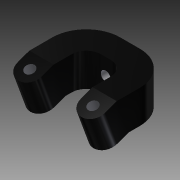
# Autodesk Inventor part: MountC
Saved by Autodesk Inventor 2015 (Build 190159000, 159)
## iProperties
Created: 2017-01-08
Part Number: MountC
Material: Generic
Document SubType Name: Modeling
Designer: Ernest
Density: 1 g/cm^3
Appearance: Default
Mass: 135.561 g
Surface Area: 237.117 cm^2
Volume: 135.561 cm^3
Author: Ernest
Autodesk Inventor part; units mm, degrees
ref_plane "YZ Plane" through (0, 0, 0) normal (1, 0, 0) x (0, 1, 0)
ref_plane "XZ Plane" through (0, 0, 0) normal (0, 1, 0) x (-1, 0, 0)
sketch "Sketch1" plane through (0, 0, 0) normal (0, 0, 1) x (1, 0, 0)
  circle A0 centre (0, 0) radius 5
  circle A1 centre (65, 0) radius 5
  circle A2 centre (0, 0) radius 12.5
  circle A3 centre (65, 0) radius 12.5
  line L0 (22.5, 9.5) -> (42.5, 9.5)
  line L1 (42.5, 9.5) -> (42.5, -10.5)
  line L2 (42.5, -10.5) -> (22.5, -10.5)
  line L3 (22.5, -10.5) -> (22.5, 9.5)
  line L4 (0, 0) -> (65, 0) construction
  line L5 (32.5, 0) -> (32.5, 40) construction
  line L6 (27.5, 40) -> (37.5, 40)
  line L7 (12.5, 0) -> (12.5, 25)
  line L8 (52.5, 0) -> (52.5, 25)
  arc A4 (27.5, 40) -> (12.5, 25) centre (27.5, 25) ccw
  arc A5 (52.5, 25) -> (37.5, 40) centre (37.5, 25) ccw
  line L9 (-12.5, 0) -> (-12.5, 30)
  line L10 (77.5, 0) -> (77.5, 30)
  line L11 (22.5, 65) -> (42.5, 65)
  arc A6 (22.5, 65) -> (-12.5, 30) centre (22.5, 30) ccw
  arc A7 (77.5, 30) -> (42.5, 65) centre (42.5, 30) ccw
  point P0 (22.5, 40)
  point P1 (42.5, 40)
  dimension "d0" = 10
  dimension "d1" = 10
  dimension "d2" = 65
  dimension "d3" = 25
  dimension "d4" = 25
  dimension "d5" = 22.5
  dimension "d6" = 22.5
  dimension "d7" = 9.5
  dimension "d8" = 10.5
  dimension "d11" = 20
  dimension "d12" = 10
  dimension "d13" = 40
  dimension "d14" = 15
  dimension "d15" = 65
  dimension "d16" = 35
  constraints: 24 end point, 12 point on circle, 12 tangent, 8 centre point, 4 horizontal, 4 point on line, 3 coincident, 3 perpendicular, 3 vertical, 2 equal radius, 2 midpoint, 2 parallel
  measures "d0" diameter of A0
  measures "d1" diameter of A1
  measures "d2" distance of A1.centre point (0, 0)
  measures "d3" diameter of A2
  measures "d4" diameter of A3
  measures "d5" distance from line of L3 point (0, 0)
  measures "d6" distance from line of L1 A1.centre
  measures "d7" distance from line of L0 point (0, 0)
  measures "d8" distance from line of point (0, 0) L2
  measures "d11" distance of point (22.5, 40) point (42.5, 40)
  measures "d12" distance of L5.end point (22.5, 40)
  measures "d13" distance of L5.start L5.end
  measures "d14" radius of A4
  measures "d15" distance from line of L11 L5.start
  measures "d16" radius of A6
extrude "Extrusion1" add sketch "Sketch1" along normal blind 34 contours A0 | A1 | A2 | A2 L9 A6 L11 A7 L10 A3 L8 A5 L6 A4 L7 | A3
ref_plane "Work Plane4" through (42.5, 65, 0) normal (0, 0.342, -0.9397) x (-1, 0, 0)
sketch "Sketch17" plane through (42.5, 65, 0) normal (0, 0.342, -0.9397) x (-1, 0, 0)
  ellipse E0 centre (42.5, -49.4513) end of major axis (30, -49.4513) minor radius 11.7462 (30, -49.4513) -> (55, -49.4513) ccw projected
  line L0 (30, -49.4513) -> (30, -25.959) projected
  ellipse E1 centre (15, -25.959) end of major axis (30, -25.959) minor radius 14.0954 (30, -25.959) -> (15, -11.8636) ccw projected
  line L1 (15, -11.8636) -> (5, -11.8636) projected
  ellipse E2 centre (5, -25.959) end of major axis (20, -25.959) minor radius 14.0954 (5, -11.8636) -> (-10, -25.959) ccw projected
  line L2 (-10, -25.959) -> (-10, -49.4513) projected
  ellipse E3 centre (-22.5, -49.4513) end of major axis (-35, -49.4513) minor radius 11.7462 (-35, -49.4513) -> (-10, -49.4513) ccw projected
  line L3 (-35, -49.4513) -> (-35, -21.2606) projected
  ellipse E4 centre (0, -21.2606) end of major axis (-35, -21.2606) minor radius 32.8892 (0, 11.6287) -> (-35, -21.2606) ccw projected
  line L4 (0, 11.6287) -> (20, 11.6287) projected
  ellipse E5 centre (20, -21.2606) end of major axis (55, -21.2606) minor radius 32.8892 (55, -21.2606) -> (20, 11.6287) ccw projected
  line L5 (55, -21.2606) -> (55, -49.4513) projected
  circle A0 centre (-22.5, -56.1975) radius 5
  circle A1 centre (42.5, -56.1975) radius 5
  circle A2 centre (-22.5, -56.1975) radius 12.5
  circle A3 centre (42.5, -56.1975) radius 12.5
  point P0 (42.5, -61.08)
  dimension "d83" = 10
  dimension "d84" = 10
  dimension "d85" = 25
  dimension "d86" = 25
  constraints: 4 centre point, 2 coincident, 8 other
  measures "d83" diameter of A0
  measures "d84" diameter of A1
  measures "d85" diameter of A2
  measures "d86" diameter of A3
extrude "Extrusion21" cut sketch "Sketch17" against normal blind 75.25 contours A1 | A0
extrude "Extrusion22" add sketch "Sketch17" against normal blind 58 contours A3 E0 | E0 A3 | A2 E3 | E3 A2
extrude "Extrusion23" cut sketch "Sketch17" against normal blind 15.9044 contours A3 E0 | E0 A3 | A2 E3 | E3 A2
sketch "Sketch19" plane through (65, 6.752, -4.2754) normal (0, 0.342, -0.9397) x (-1, 0, 0)
  circle A0 centre (0, 0) radius 5 projected
  circle A1 centre (0, 0) radius 12.5 projected
  circle A2 centre (65, 0) radius 5 projected
  circle A3 centre (65, 0) radius 12.5 projected
  line L0 (-12.5, 0) -> (-17.2667, 0)
  line L1 (-17.2667, 0) -> (-17.2667, -28.7026)
  line L2 (-17.2667, -28.7026) -> (21.0012, -28.7026)
  line L3 (21.0012, -28.7026) -> (21.0012, 0)
  line L4 (21.0012, 0) -> (12.5, 0)
  line L5 (52.5, 0) -> (49.0235, 0)
  line L6 (49.0235, 0) -> (49.0235, -27.0388)
  line L7 (49.0235, -27.0388) -> (85.6276, -27.0388)
  line L8 (85.6276, -27.0388) -> (85.6276, 0)
  line L9 (85.6276, 0) -> (77.5, 0)
  circle A4 centre (0, 0) radius 12.5
  circle A5 centre (65, 0) radius 12.5
  line L10 (-12.5, 0) -> (-12.5, 6.7462) projected
  line L11 (-12.5, -4.8825) -> (-12.5, 0) projected
  line L12 (-12.5, -4.8825) -> (-12.5, 0) projected
  line L13 (-12.5, 0) -> (-12.5, 23.3083) projected
  line L14 (-12.5, 23.3083) -> (-12.5, 34.9369) projected
  line L15 (-12.5, 6.7462) -> (-12.5, 34.9369) projected
  line L16 (77.5, 34.9369) -> (77.5, 6.7462) projected
  line L17 (77.5, 23.3083) -> (77.5, 34.9369) projected
  line L18 (77.5, 23.3083) -> (77.5, 0) projected
  line L19 (77.5, 0) -> (77.5, -4.8825) projected
  line L20 (77.5, -4.8825) -> (77.5, 0) projected
  line L21 (77.5, 0) -> (77.5, 6.7462) projected
  circle A6 centre (0, 0) radius 5 projected
  line L22 (12.5, 30.2385) -> (12.5, 6.7462) projected
  line L23 (12.5, 18.6098) -> (12.5, 30.2385) projected
  line L24 (12.5, 18.6098) -> (12.5, 0) projected
  line L25 (12.5, 0) -> (12.5, -4.8825) projected
  line L26 (12.5, -4.8825) -> (12.5, 0) projected
  line L27 (12.5, 0) -> (12.5, 6.7462) projected
  line L28 (52.5, 0) -> (52.5, 6.7462) projected
  line L29 (52.5, -4.8825) -> (52.5, 0) projected
  line L30 (52.5, -4.8825) -> (52.5, 0) projected
  line L31 (52.5, 0) -> (52.5, 18.6098) projected
  line L32 (52.5, 18.6098) -> (52.5, 30.2385) projected
  line L33 (52.5, 6.7462) -> (52.5, 30.2385) projected
  line L34 (-12.5, 0) -> (-12.5, 23.3083) projected
  line L35 (-12.5, 15.1562) -> (-12.5, -17.0681)
  line L36 (-12.5, -17.0681) -> (12.5, -17.0681)
  line L37 (12.5, -17.0681) -> (12.5, 15.1562)
  line L38 (12.5, 18.6098) -> (12.5, 0) projected
  line L39 (12.5, 15.1562) -> (-12.5, 15.1562)
  line L40 (52.5, 0) -> (52.5, 18.6098) projected
  line L41 (52.5, 15.1562) -> (52.5, -18.9753)
  line L42 (52.5, -18.9753) -> (77.5, -18.9753)
  line L43 (77.5, -18.9753) -> (77.5, 15.1562)
  line L44 (77.5, 23.3083) -> (77.5, 0) projected
  line L45 (77.5, 15.1562) -> (52.5, 15.1562)
  point P0 (65, -4.8825)
  point P1 (-12.5, 12.5)
  point P2 (-12.5, 5.9839)
  point P3 (77.5, 5.9839)
  point P4 (77.5, 12.5)
  point P5 (12.5, 5.9839)
  point P6 (12.5, 12.5)
  point P7 (52.5, 12.5)
  point P8 (52.5, 5.9839)
  constraints: 36 end point, 13 point on line, 10 perpendicular, 2 centre point, 2 coincident, 2 point on circle, 1 concentric, 1 horizontal
extrude "Extrusion29" add sketch "Sketch19" against normal blind 36.087 contours L25 L37 L36 L35 L11 A1 | A1 L10 L13 L39 L22 L24 | L19 L43 L42 L41 L29 A3 | A3 L28 L31 L45 L16 L18
extrude "Extrusion25" cut sketch "Sketch19" against normal blind 107.25 contours L25 L37 L36 L35 L11 A1 | L4 L3 L2 L1 L0 L11 L35 L36 L37 L25 | L19 L43 L42 L41 L29 A3 | L9 L8 L7 L6 L5 L29 L41 L42 L43 L19
sketch "Sketch20" plane through (22.5, 65, 0) normal (0, 1, 0) x (1, 0, 0)
  line L0 (20, 0) -> (0, 0) projected
  line L1 (0, 0) -> (0, -34) projected
  line L2 (20, -34) -> (0, -34) projected
  line L3 (20, 0) -> (20, -34) projected
  circle A0 centre (10, -17) radius 5
  point P0 (-22.5, 0)
  dimension "d97" = 10
  dimension "d98" = 20
  dimension "d99" = 34
  dimension "d100" = 17
  dimension "d101" = 10
  constraints: 1 centre point
  measures "d97" diameter of A0
  measures "d98" distance of L0.start L0.end
  measures "d99" distance of L0.end L1.end
  measures "d100" distance from line of L0 A0.centre
  measures "d101" distance from line of L1 A0.centre
extrude "Extrusion26" cut sketch "Sketch20" against normal blind 107.25 contours A0
sketch "Sketch24" plane through (77.5, 30, 34) normal (1, 0, 0) x (0, 0, -1)
  line L0 (4.3647, -35.5905) -> (38.2754, -23.248) projected
  line L1 (34, -11.5014) -> (38.2754, -23.248) projected
  line L2 (34, -11.5014) -> (34, 0) projected
  line L3 (34, 0) -> (0, 0) projected
  line L4 (0, -21.0502) -> (0, 0) projected
  line L5 (0, -21.0502) -> (-0.819, -21.3483) projected
  line L6 (0, -23.5985) -> (-0.819, -21.3483) projected
  line L7 (0, -30) -> (0, -23.5985) projected
  line L8 (2.33, -30) -> (0, -30) projected
  line L9 (4.3647, -35.5905) -> (2.33, -30) projected
  line L10 (-5.5567, -25.8994) -> (2.9938, -49.3917) projected
  line L11 (4.3647, -35.5905) -> (3.379, -32.8821) projected
  line L12 (0, -33.478) -> (3.379, -32.8821) projected
  line L13 (0, -33.478) -> (0, -33.478) projected
  line L14 (3.379, -32.8821) -> (0, -33.478) projected
  line L15 (3.379, -32.8821) -> (4.3647, -35.5905) projected
  line L16 (38.2754, -23.248) -> (4.3647, -35.5905) projected
  line L17 (38.2754, -23.248) -> (38.2754, -23.248) projected
  line L18 (4.3647, -35.5905) -> (38.2754, -23.248) projected
  line L19 (0, -19.3385) -> (0, -23.5985)
  line L20 (0, -23.5985) -> (9.2627, -49.0475)
  line L21 (2.33, -30) -> (3.379, -32.8821) projected
  line L22 (9.2627, -49.0475) -> (-1.2815, -52.8852)
  line L23 (-1.2815, -52.8852) -> (-12.2937, -22.6295)
  line L24 (0, -19.3385) -> (-12.2937, -22.6295)
  point P0 (34, -30)
  constraints: 10 end point, 2 collinear, 2 perpendicular, 1 point on line
extrude "Extrusion31" cut sketch "Sketch24" against normal blind 97.087 contours L20 L22 L23 L24 L4 L5 L6 L7 L8 L9 | L8 L7 L20 | L6 L5 L19
equation "\"d12\" = 0.5 * d11"
equation "\"d15\" = d13 + d3"
equation "\"d100\" = 0.5 * d99"
equation "\"d101\" = 0.5 * d98"
body "Solid1"
